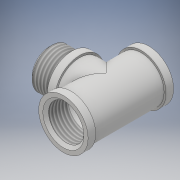
# Autodesk Inventor part: Инж_граф_2
Saved by Autodesk Inventor 2019.3 (Build 233278000, 278)
## iProperties
Created: 2020-03-31
Part Number: Инж_граф_2
Material: Типовые
Document SubType Name: Modeling
Designer: Diana
Density: 1 g/cm^3
Appearance: По умолчанию
Mass: 12.694 g
Surface Area: 89.0778 cm^2
Volume: 12.694 cm^3
Author: Diana
Autodesk Inventor part; units mm, degrees
ref_plane "YZ Plane" through (0, 0, 0) normal (1, 0, 0) x (0, 1, 0)
ref_plane "XZ Plane" through (0, 0, 0) normal (0, 1, 0) x (-1, 0, 0)
ref_plane "XY Plane" through (0, 0, 0) normal (0, 0, 1) x (1, 0, 0)
sketch "Эскиз1" plane through (0, 0, 0) normal (0, 0, 1) x (1, 0, 0)
  circle A0 centre (0, 0) radius 12
  dimension "d0" = 24
  constraints: 1 centre point, 1 coincident
  measures "d0" diameter of A0
extrude "Выдавливание1" add sketch "Эскиз1" along normal mid plane 37
sketch "Эскиз7" plane through (0, 0, 18.5) normal (0, 0, 1) x (1, 0, 0)
  circle A0 centre (0, 0) radius 13
  dimension "d27" = 26
  constraints: 1 centre point, 1 coincident
  measures "d27" diameter of A0
extrude "Выдавливание7" add sketch "Эскиз7" along normal blind 4
mirror "Зеркальное отражение1" about plane through (0, 0, 0) normal (0, 0, 1) of "Выдавливание7"
sketch "Эскиз8" plane through (0, 0, 0) normal (1, 0, 0) x (0, 1, 0)
  circle A0 centre (0, 0) radius 12
  dimension "d30" = 24
  constraints: 1 centre point, 1 coincident
  measures "d30" diameter of A0
extrude "Выдавливание8" add sketch "Эскиз8" against normal blind 14
sketch "Эскиз9" plane through (-14, 0, 0) normal (-1, 0, 0) x (0, 0, 1)
  circle A0 centre (0, 0) radius 13
  dimension "d33" = 26
  constraints: 1 centre point, 1 coincident
  measures "d33" diameter of A0
extrude "Выдавливание9" add sketch "Эскиз9" along normal blind 4
sketch "Эскиз10" plane through (-18, 0, 0) normal (-1, 0, 0) x (0, 0, 1)
  circle A0 centre (0, 0) radius 10.4775
  dimension "d36" = 20.955
  constraints: 1 centre point, 1 coincident
  measures "d36" diameter of A0
extrude "Выдавливание10" add sketch "Эскиз10" along normal blind 12
thread "Резьба1" size "G20.955x1.814" designation "G 1/2" class "A" standard "ISO Pipe Threads" length 11
sketch "Эскиз11" plane through (0, 0, 22.5) normal (0, 0, 1) x (1, 0, 0)
  circle A0 centre (0, 0) radius 9.3155
  dimension "d41" = 18.631
  constraints: 1 centre point, 1 coincident
  measures "d41" diameter of A0
extrude "Выдавливание11" cut sketch "Эскиз11" against normal through all
thread "Резьба2" size "G20.955x1.814" designation "G 1/2" standard "ISO Pipe Threads" length 12
thread "Резьба3" size "G20.955x1.814" designation "G 1/2" standard "ISO Pipe Threads" length 12
sketch "Эскиз12" plane through (-30, 0, 0) normal (-1, 0, 0) x (0, 0, 1)
  circle A0 centre (0, 0) radius 7.5
  dimension "d48" = 15
  constraints: 1 centre point, 1 coincident
  measures "d48" diameter of A0
extrude "Выдавливание12" cut sketch "Эскиз12" against normal up to next
chamfer "Фаска5" distance 1.5 angle 45 1 edges at (-30, 0, -10.4775)
chamfer "Фаска6" distance 1.5 angle 45 1 edges at (-9.3155, 0, -22.5)
chamfer "Фаска7" distance 1.5 angle 45 1 edges at (-9.3155, 0, 22.5)
